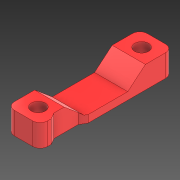
# Autodesk Inventor part: CH_01_0033_syringe_pump_nut_mount
Saved by Autodesk Inventor 2022 (Build 260153000, 153)
## iProperties
Created: 2022-04-22
Part Number: CH_01_0033_syringe_pump_nut_mount
Material: ABS Plastic
Document SubType Name: Modeling
Designer: Tomasz Krakowski
Density: 1.06 g/cm^3
Appearance: Light Red
Author: Tomasz Krakowski
Autodesk Inventor part; units mm, degrees
ref_plane "YZ Plane" through (0, 0, 0) normal (1, 0, 0) x (0, 1, 0)
ref_plane "XZ Plane" through (0, 0, 0) normal (0, 1, 0) x (-1, 0, 0)
ref_plane "XY Plane" through (0, 0, 0) normal (0, 0, 1) x (1, 0, 0)
sketch "Sketch1" plane through (0, 0, 0) normal (0, 1, 0) x (-1, 0, 0)
  line L0 (-2.5, 18) -> (2.5, 18)
  line L1 (4.5, 16) -> (4.5, -16)
  line L2 (2.5, -18) -> (-2.5, -18)
  line L3 (-4.5, -16) -> (-4.5, 16)
  line L4 (-4.5, 18) -> (4.5, -18) construction
  line L5 (4.5, 18) -> (-4.5, -18) construction
  circle A0 centre (0, 14) radius 1.9
  line L6 (0, 14) -> (0, -14) construction
  circle A1 centre (0, -14) radius 1.9
  arc A2 (4.5, 16) -> (2.5, 18) centre (2.5, 16) ccw
  arc A3 (2.5, -18) -> (4.5, -16) centre (2.5, -16) ccw
  arc A4 (-4.5, -16) -> (-2.5, -18) centre (-2.5, -16) ccw
  arc A5 (-2.5, 18) -> (-4.5, 16) centre (-2.5, 16) ccw
  point P0 (0, 0)
  point P1 (0, 0)
  dimension "d0" = 3.8
  dimension "d1" = 28
  dimension "d2" = 36
  dimension "d3" = 9
  dimension "d4" = 2
  dimension "d5" = 2
  dimension "d6" = 2
  constraints: 14 end point, 8 point on circle, 8 point on line, 8 tangent, 6 centre point, 5 midpoint, 2 equal radius, 2 parallel, 1 coincident, 1 horizontal, 1 perpendicular, 1 vertical
  measures "d0" diameter of A0
  measures "d1" distance of L6.end L6.start
  measures "d2" distance between parallel lines of L2 L0
  measures "d3" distance between parallel lines of L1 L3
  measures "d4" radius of A2
  measures "d5" radius of A3
  measures "d6" radius of A4
extrude "Extrusion1" add sketch "Sketch1" along normal blind 6
sketch "Sketch2" plane through (4.5, 0, 16) normal (1, 0, 0) x (0, 0, -1)
  line L0 (32, 6) -> (0, 6) construction
  line L1 (5.5, 6) -> (10.267, 2)
  line L2 (10.267, 2) -> (16, 2)
  line L3 (16, 0) -> (16, 6) construction
  line L4 (16, 2) -> (16, 6)
  line L5 (5.5, 6) -> (16, 6)
  line L6 (0, 0) -> (32, 0) projected
  line L7 (26.5, 6) -> (21.733, 2)
  line L8 (21.733, 2) -> (16, 2)
  line L9 (26.5, 6) -> (16, 6)
  dimension "d9" = 2
  dimension "d10" = 10.5
  dimension "d11" = 40
  constraints: 16 end point, 2 symmetric about line, 1 collinear, 1 horizontal, 1 midpoint, 1 parallel, 1 perpendicular, 1 point on line
  measures "d9" distance between parallel lines of L6 L2
  measures "d10" distance from line of L4 L1.start
  measures "d11" angle of L0 L1
extrude "Extrusion2" cut sketch "Sketch2" against normal through all
sketch "Sketch3" plane through (0, 0, 0) normal (0, -1, 0) x (1, 0, 0)
  line L0 (4.5, 16) -> (4.5, -16) construction
  line L1 (4.5, 15) -> (3.5, 13.2679)
  line L2 (3.5, 13.2679) -> (3.5, 6.7321)
  line L3 (3.5, 6.7321) -> (4.5, 5)
  line L4 (4.5, 15) -> (4.5, 5)
  line L5 (-2.5, 18) -> (2.5, 18) projected
  point P0 (0, 0)
  dimension "d14" = 150
  dimension "d15" = 150
  dimension "d16" = 1
  dimension "d17" = 3
  dimension "d18" = 10
  constraints: 8 end point, 2 point on line, 1 collinear, 1 parallel
  measures "d14" angle of L0 L1
  measures "d15" angle of L0 L3
  measures "d16" distance between parallel lines of L0 L2
  measures "d17" distance from line of L5 L1.start
  measures "d18" distance of L3.end L1.start
extrude "Extrusion3" cut sketch "Sketch3" against normal through all
body "Solid1"
